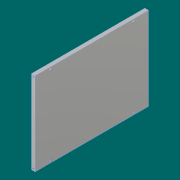
# Autodesk Inventor part: leftSide
Saved by Autodesk Inventor 2017 (Build 210142000, 142)
## iProperties
Created: 2015-10-13
Part Number: leftSide
Material: Aluminum 6061
Document SubType Name: Modeling
Designer: Sawaiz
Density: 2.7 g/cm^3
Appearance: Aluminum - Flat
Author: Sawaiz
Autodesk Inventor part; units mm, degrees
ref_plane "YZ Plane" through (0, 0, 0) normal (1, 0, 0) x (0, 1, 0)
ref_plane "XZ Plane" through (0, 0, 0) normal (0, 1, 0) x (-1, 0, 0)
ref_plane "XY Plane" through (0, 0, 0) normal (0, 0, 1) x (1, 0, 0)
sketch "Sketch1" plane through (0, 0, 0) normal (0, 1, 0) x (-1, 0, 0)
  line L0 (-95.25, 69.85) -> (95.25, 69.85)
  line L1 (95.25, 69.85) -> (95.25, -69.85)
  line L2 (95.25, -69.85) -> (-95.25, -69.85)
  line L3 (-95.25, -69.85) -> (-95.25, 69.85)
  line L4 (-95.25, 69.85) -> (95.25, -69.85) construction
  line L5 (95.25, 69.85) -> (-95.25, -69.85) construction
  point P0 (0, 0)
  dimension "d0" = 190.5
  dimension "d1" = 139.7
  constraints: 12 end point, 2 midpoint, 2 parallel, 1 horizontal, 1 perpendicular
  measures "d0" distance of L1.end L2.end
  measures "d1" distance of L0.end L1.end
extrude "Extrusion1" add sketch "Sketch1" along normal blind 6.35
sketch "Sketch9" plane through (95.25, 0, 69.85) normal (1, 0, 0) x (0, 0, -1)
  line L0 (139.7, 0) -> (0, 0) projected
  line L1 (139.7, 0) -> (139.7, 6.35) projected
  line L2 (0, 6.35) -> (139.7, 6.35) projected
  line L3 (0, 0) -> (0, 6.35) projected
  point P0 (69.85, 0)
  point P1 (3.175, 3.175)
  dimension "d45" = 3.175
  dimension "d46" = 3.175
  measures "d45" distance from line of L0 point (3.175, 3.175)
  measures "d46" distance from line of L3 point (3.175, 3.175)
hole "Hole3" at (95.25, 3.175, 66.675) direction (-1, 0, 0) diameter 2.159 depth 8.8646 tip angle 118
mirror "Mirror5" about plane through (0, 0, 0) normal (0, 0, 1) of "Hole3"
mirror "Mirror6" about plane through (0, 0, 0) normal (1, 0, 0) of "Hole3", "Mirror5"
sketch "Sketch11" plane through (0, 0, 0) normal (0, -1, 0) x (1, 0, 0)
  line L0 (95.25, 69.85) -> (-95.25, 69.85) projected
  line L1 (-95.25, 69.85) -> (-95.25, -69.85) projected
  line L2 (-95.25, -69.85) -> (95.25, -69.85) projected
  line L3 (95.25, -69.85) -> (95.25, 69.85) projected
  point P0 (0, 0)
  point P1 (-69.85, 66.675)
  dimension "d61" = 25.4
  dimension "d62" = 3.175
  measures "d61" distance from line of L1 point (-69.85, 66.675)
  measures "d62" distance from line of L0 point (-69.85, 66.675)
hole "Hole4" at (-69.85, 0, 66.675) direction (0, 1, 0) diameter 3.2766 end through all countersink diameter 5.715 countersink angle 82 clearance for "Flat Head Machine Screw (82)" size "#4" standard "Ansi Unified Screw Threads"
mirror "Mirror7" about plane through (0, 0, 0) normal (1, 0, 0) of "Hole4"
mirror "Mirror8" about plane through (0, 0, 0) normal (0, 0, 1) of "Hole4", "Mirror7"
equation "\"d0\" = depth"
equation "\"d1\" = height + 2 * plasticThickness"
equation "\"d2\" = caseThickness"
equation "\"d45\" = 0.5 * caseThickness"
equation "\"d46\" = 0.5 * caseThickness"
equation "\"d61\" = 4 * caseThickness"
equation "\"d62\" = 0.5 * caseThickness"
equation "\"acrylicThickness\" = 9.525"
equation "\"depth\" = 190.5"
equation "\"height\" = 127"
equation "\"fresnelThickness\" = 0.254"
equation "\"focalLength\" = 152.4"
equation "\"centerThickness\" = 1.27"
equation "\"sensorHolderDepth\" = 19.05"
equation "\"internalAcrylicThickness\" = 6.35"
equation "\"frameAcrylicThickness\" = 9.525"
equation "\"width\" = 127"
equation "\"mirrorAngle\" = 5deg"
equation "\"detectorWidth\" = 52"
equation "\"detectorHeight\" = 52"
equation "\"mirrorThickness\" = 3.175"
equation "\"ior\" = 1.49"
equation "\"fresnelAngle\" = 90deg"
equation "\"fresnelEffectiveDiameter\" = 152.4"
equation "\"oRingWidth\" = 1.5875"
equation "\"aerogelClearence\" = 3.175"
equation "\"backplaneHoleOffsett\" = 6.35"
equation "\"backplanePCBHeight\" = 76.2"
equation "\"backplanePCBWidth\" = 76.2"
equation "\"backplanePostionOffsett\" = 12.7"
equation "\"moduleSlotClearence\" = 0.79375"
equation "\"plasticThickness\" = 6.35"
equation "\"aerogelHolderDepth\" = 36.5125"
equation "\"caseThickness\" = 6.35"
equation "\"alignmantGrooveDepth\" = 1.5875"
equation "\"alignmentGrooveDepth\" = 1.5875"
equation "\"alignmentGrooveClearance\" = 0.1016"
equation "\"frontPanelThickness\" = 2.38125"
body "Solid1"
